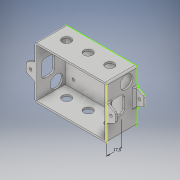
# Autodesk Inventor part: Contenedor del Arduino v1.1
Saved by Autodesk Inventor 2019 (Build 230136000, 136)
## iProperties
Created: 2018-07-23
Part Number: Contenedor del Arduino v1.1
Material: Genérico
Document SubType Name: Modeling
Designer: Francisco
Density: 1 g/cm^3
Appearance: Valor por defecto
Author: Francisco
Autodesk Inventor part; units mm, degrees
ref_plane "YZ Plane" through (0, 0, 0) normal (1, 0, 0) x (0, 1, 0)
ref_plane "XZ Plane" through (0, 0, 0) normal (0, 1, 0) x (-1, 0, 0)
sketch "Base" plane through (0, 0, 0) normal (0, 0, 1) x (1, 0, 0)
  line L0 (-41.5, -30) -> (41.5, -30)
  line L1 (41.5, -30) -> (41.5, -11.2361)
  line L2 (41.5, 30) -> (-41.5, 30)
  line L3 (-41.5, -30) -> (41.5, 30) construction
  line L4 (41.5, -30) -> (-41.5, 30) construction
  line L5 (-39.5, -28) -> (39.5, -28)
  line L6 (39.5, -28) -> (39.5, 28)
  line L7 (39.5, 28) -> (-39.5, 28)
  line L8 (-39.5, 28) -> (-39.5, -28)
  circle A0 centre (-30, -18.5) radius 1.35
  circle A1 centre (30, -18.5) radius 1.35
  circle A2 centre (0, 18.5) radius 1.35
  line L9 (51.5, 3.7639) -> (51.5, -3.7639)
  line L10 (41.5, 5) -> (51.5, -5) construction
  line L11 (51.5, 5) -> (41.5, -5) construction
  line L12 (42.6056, -9.4472) -> (50.3944, -5.5528)
  line L13 (50.3944, 5.5528) -> (42.6056, 9.4472)
  arc A3 (51.5, 3.7639) -> (50.3944, 5.5528) centre (49.5, 3.7639) ccw
  arc A4 (50.3944, -5.5528) -> (51.5, -3.7639) centre (49.5, -3.7639) ccw
  arc A5 (42.6056, -9.4472) -> (41.5, -11.2361) centre (43.5, -11.2361) ccw
  line L14 (41.5, 11.2361) -> (41.5, 30)
  arc A6 (41.5, 11.2361) -> (42.6056, 9.4472) centre (43.5, 11.2361) ccw
  line L15 (-41.5, -30) -> (-41.5, -11.2361)
  line L16 (-39.5, -28) -> (-39.5, 28)
  line L17 (-51.5, 3.7639) -> (-51.5, -3.7639)
  line L18 (-41.5, 5) -> (-51.5, -5) construction
  line L19 (-51.5, 5) -> (-41.5, -5) construction
  line L20 (-42.6056, -9.4472) -> (-50.3944, -5.5528)
  line L21 (-50.3944, 5.5528) -> (-42.6056, 9.4472)
  arc A7 (-50.3944, 5.5528) -> (-51.5, 3.7639) centre (-49.5, 3.7639) ccw
  arc A8 (-51.5, -3.7639) -> (-50.3944, -5.5528) centre (-49.5, -3.7639) ccw
  arc A9 (-41.5, -11.2361) -> (-42.6056, -9.4472) centre (-43.5, -11.2361) ccw
  line L22 (-41.5, 11.2361) -> (-41.5, 30)
  arc A10 (-42.6056, 9.4472) -> (-41.5, 11.2361) centre (-43.5, 11.2361) ccw
  line L23 (41.5, 11.2361) -> (41.5, -11.2361)
  line L24 (-41.5, -11.2361) -> (-41.5, 11.2361)
  circle A11 centre (-46.5, 0) radius 1.35
  circle A12 centre (46.5, 0) radius 1.35
  circle A13 centre (0, 18.5) radius 1.6
  circle A14 centre (30, -18.5) radius 1.6
  circle A15 centre (-30, -18.5) radius 1.6
  circle A16 centre (-46.5, 0) radius 1.6
  circle A17 centre (46.5, 0) radius 1.6
  point P0 (0, 0)
  point P1 (41.5, 10)
  point P2 (-41.5, 10)
  point P3 (-41.5, -10)
  point P4 (-41.5, 10)
  dimension "d0" = 83
  dimension "d1" = 60
  dimension "d5" = 2.7
  dimension "d6" = 9.5
  dimension "d8" = 2.7
  dimension "d9" = 5
  dimension "d10" = 10
  dimension "d11" = 10
  dimension "d14" = 2
  dimension "d15" = 2
  dimension "d16" = 2.7
  dimension "d17" = 2.7
  dimension "d63" = 3.2
  dimension "d64" = 3.2
  dimension "d65" = 3.2
  dimension "d66" = 3.2
  dimension "d67" = 3.2
  constraints: 50 end point, 18 centre point, 16 point on circle, 14 point on line, 10 coincident, 8 tangent, 6 midpoint, 4 parallel, 2 equal radius, 2 perpendicular, 1 horizontal, 1 vertical, 2 other
  measures "d0" distance of L2.end L2.start
  measures "d1" distance of L2.start L0.end
  measures "d5" diameter of A0
  measures "d6" distance from line of L7 point (0, 18.5)
  measures "d8" diameter of A2
  measures "d9" distance from line of L1 point (46.5, 0)
  measures "d10" distance of L10.end L11.end
  measures "d11" distance of L11.start L10.end
  measures "d14" radius of A3
  measures "d15" radius of A6
  measures "d16" diameter of A11
  measures "d17" diameter of A12
  measures "d63" diameter of A13
  measures "d64" diameter of A14
  measures "d65" diameter of A15
  measures "d66" diameter of A16
  measures "d67" diameter of A17
extrude "Extrusión1" add sketch "Base" along normal blind 2 contours L8 L7 L6 L5 | A13 | A14 | A15
extrude "Extrusión2" add sketch "Base" along normal blind 2 contours A9 L20 A8 L17 A7 L21 A10 L24 | L23 A6 L13 A3 L9 A4 L12 A5 | A16 | A17
extrude "Extrusión3" cut sketch "Base" along normal blind 35 contours L15 L24 L22 L2 L14 L23 L1 L0
extrude "Extrusión4" add sketch "Base" along normal blind 35 contours L15 L24 L22 L2 L14 L23 L1 L0
sketch "Boceto2" plane through (-41.5, 30, 0) normal (0, 1, 0) x (1, 0, 0)
  line L0 (41.5, 0) -> (41.5, -35)
  line L1 (2, -35) -> (81, -35) projected
  line L2 (83, 0) -> (0, 0) projected
  circle A0 centre (16.5, -14.9) radius 5
  circle A1 centre (66.5, -14.9) radius 5
  circle A2 centre (41.5, -14.9) radius 5
  dimension "d26" = 14.9
  dimension "d27" = 25
  dimension "d28" = 10
  dimension "d29" = 10
  constraints: 3 centre point, 2 end point, 1 coincident, 1 midpoint, 1 point on line, 1 symmetric about line, 1 other
  measures "d26" distance from line of L2 point (16.5, -14.9)
  measures "d27" distance from line of L0 point (16.5, -14.9)
  measures "d28" diameter of A0
  measures "d29" diameter of A2
extrude "Extrusión5" cut sketch "Boceto2" against normal blind 70
sketch "Boceto3" plane through (41.5, 11.2361, 0) normal (1, 0, 0) x (0, 0, -1)
  line L0 (-2, -39.2361) -> (-35, -39.2361) projected
  line L1 (-2, -15) -> (-2, -7.4721) projected
  line L2 (0, 0) -> (0, 18.7639) projected
  line L3 (-18.5, -21.2361) -> (-25.5, -21.2361)
  line L4 (-29.5, -17.2361) -> (-29.5, -5.2361)
  line L5 (-25.5, -1.2361) -> (-18.5, -1.2361)
  line L6 (-14.5, -5.2361) -> (-14.5, -17.2361)
  line L7 (-14.5, -21.2361) -> (-29.5, -1.2361) construction
  line L8 (-29.5, -21.2361) -> (-14.5, -1.2361) construction
  arc A0 (-29.5, -17.2361) -> (-25.5, -21.2361) centre (-25.5, -17.2361) ccw
  arc A1 (-18.5, -21.2361) -> (-14.5, -17.2361) centre (-18.5, -17.2361) ccw
  arc A2 (-14.5, -5.2361) -> (-18.5, -1.2361) centre (-18.5, -5.2361) ccw
  arc A3 (-25.5, -1.2361) -> (-29.5, -5.2361) centre (-25.5, -5.2361) ccw
  circle A4 centre (-12, 8.7639) radius 7.5
  point P0 (0, -11.2361)
  point P1 (-22, -11.2361)
  dimension "d32" = 28
  dimension "d33" = 48
  dimension "d34" = 20
  dimension "d35" = 12
  dimension "d36" = 15
  dimension "d37" = 20
  dimension "d38" = 4
  dimension "d39" = 15
  constraints: 12 end point, 8 point on circle, 8 point on line, 8 tangent, 5 centre point, 3 equal radius, 2 midpoint, 2 parallel, 1 coincident, 1 horizontal, 1 perpendicular
  measures "d32" distance from line of L0 point (-22, -11.236)
  measures "d33" distance from line of L0 point (-12, 8.764)
  measures "d34" distance from line of L1 point (-22, -11.236)
  measures "d35" distance from line of L2 point (-12, 8.764)
  measures "d36" distance of L7.end L8.end
  measures "d37" distance of L8.start L7.end
  measures "d38" radius of A0
  measures "d39" diameter of A4
extrude "Extrusión6" cut sketch "Boceto3" against normal blind 10
sketch3d "Boceto 3D1"
pattern_circular "Patrón circular1" count 2 over 360 about axis through (0, 0, 99.8627) along (0, 0, -1) of "Extrusión6"
sketch "Boceto4" plane through (41.5, 11.2361, 0) normal (1, 0, 0) x (0, 0, -1)
  line L0 (-35, -41.2361) -> (-35, 18.7639) projected
  point P0 (0, -11.2361)
  point P1 (-17.5, -25.9654)
  dimension "d45" = 17.5
  measures "d45" distance from line of L0 point (-17.5, -25.965)
ref_plane "Plano de trabajo1" through (41.5, -14.7294, 17.5) normal (0, 0, 1) x (1, 0, 0)
mirror "Simetría1" about plane through (41.5, -14.7294, 17.5) normal (0, 0, 1) of "Extrusión2"
chamfer "Chaflán1" distance 1.7 angle 63 1 edges at (41.5, 0, 33) measured on face at (43.0002, 0, 33)
mirror "Simetría2" about plane through (41.5, -14.7294, 17.5) normal (0, 0, 1) of "Extrusión2", "Simetría1", "Chaflán1"
chamfer "Chaflán2" distance 1.7 angle 63 1 edges at (-41.5, 0, 33) measured on face at (-43.0002, 0, 33)
chamfer "Chaflán3" distance 1.7 angle 63 1 edges at (-41.5, 0, 2) measured on face at (-43.0002, 0, 2)
fillet "Empalme1" radius 2 4 edges at (-41.5, 30, 17.5) (41.5, 30, 17.5) (41.5, -30, 17.5) (-41.5, -30, 17.5)
hole "Agujero2" at (0, 18.5, 0) at (-30, -18.5, 0) at (-46.5, 0, 0) at (30, -18.5, 0) at (46.5, 0, 0) direction (0, 0, 1) diameter 3.2 depth 23.25 tip angle 118
extrude "Extrusión8" cut sketch "Base" along normal blind 94.8 contours A16 | A17
